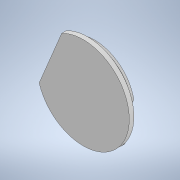
# Autodesk Inventor part: cap2
Saved by Autodesk Inventor 2020 (Build 240168000, 168)
## iProperties
Created: 2022-10-19
Part Number: cap2
Material: Типовые
Document SubType Name: Modeling
Designer: zigma
Density: 1 g/cm^3
Appearance: По умолчанию
Author: zigma
Autodesk Inventor part; units mm, degrees
ref_plane "YZ Plane" through (0, 0, 0) normal (1, 0, 0) x (0, 1, 0)
ref_plane "XZ Plane" through (0, 0, 0) normal (0, 1, 0) x (-1, 0, 0)
ref_plane "XY Plane" through (0, 0, 0) normal (0, 0, 1) x (1, 0, 0)
sketch "Эскиз1" plane through (0, 0, 0) normal (0, 0, 1) x (1, 0, 0)
  line L0 (-14.0097, -7.3348) -> (-16.3175, -6.3736)
  line L1 (-16.3175, -6.3736) -> (-14.0097, -7.3348)
  line L2 (17.7899, 2.7423) -> (-9.8124, 2.7423)
  line L3 (-14.0097, -7.3348) -> (-9.8124, 2.7423)
  line L4 (-9.8124, 2.7423) -> (17.7899, 2.7423)
  line L5 (-16.3175, -6.3736) -> (-6.7051, 16.7046)
  line L6 (-16.3175, -6.3736) -> (-6.7051, 16.7046)
  line L7 (-14.0257, -14.2577) -> (-10.5192, -14.2577)
  line L8 (-14.0257, -14.2577) -> (-10.5192, -14.2577)
  line L9 (-10.5192, -14.2577) -> (-10.5192, -12.2577)
  line L10 (-10.5192, -14.2577) -> (-10.5192, -12.2577)
  line L11 (-10.5192, -12.2577) -> (-12.5192, -12.2577)
  line L12 (-10.5192, -12.2577) -> (-12.5192, -12.2577)
  line L13 (-12.5192, -12.2577) -> (-12.5192, -10.2577)
  line L14 (-12.5192, -12.2577) -> (-12.5192, -10.2577)
  line L15 (-12.5192, -10.2577) -> (-9.4474, -10.2577)
  line L16 (-12.5192, -10.2577) -> (-9.4474, -10.2577)
  line L17 (-9.4474, -10.2577) -> (-6.5, 0.7423)
  line L18 (-9.4474, -10.2577) -> (-6.5, 0.7423)
  line L19 (-6.5, 0.7423) -> (6.5, 0.7423)
  line L20 (-6.5, 0.7423) -> (6.5, 0.7423)
  line L21 (9.4474, -10.2577) -> (12.5192, -10.2577)
  line L22 (6.5, 0.7423) -> (9.4474, -10.2577)
  line L23 (9.4474, -10.2577) -> (12.5192, -10.2577)
  line L24 (12.5192, -10.2577) -> (12.5192, -12.2577)
  line L25 (12.5192, -10.2577) -> (12.5192, -12.2577)
  line L26 (10.5192, -12.2577) -> (10.5192, -14.2577)
  line L27 (12.5192, -12.2577) -> (10.5192, -12.2577)
  line L28 (10.5192, -12.2577) -> (10.5192, -14.2577)
  line L29 (10.5192, -14.2577) -> (14.0257, -14.2577)
  arc A0 (17.7899, 2.7423) -> (-6.7051, 16.7046) centre (0, 0) ccw
  arc A1 (17.7899, 2.7423) -> (-6.7051, 16.7046) centre (0, 0) ccw
  arc A2 (17.5551, 2.9423) -> (-6.5528, 16.5499) centre (0, 0) ccw
  line L30 (17.5551, 2.9423) -> (-9.9457, 2.9423)
  line L31 (-14.1174, -7.0733) -> (-9.9457, 2.9423)
  line L32 (-16.056, -6.2659) -> (-6.5528, 16.5499)
  line L33 (-14.1174, -7.0733) -> (-16.056, -6.2659)
  arc A3 (-14.0257, -14.2577) -> (14.0257, -14.2577) centre (0, 0) ccw
  line L34 (13.5283, -14.4577) -> (10.3192, -14.4577)
  line L35 (10.3192, -12.0577) -> (10.3192, -14.4577)
  line L36 (12.3192, -12.0577) -> (10.3192, -12.0577)
  line L37 (12.3192, -10.4577) -> (12.3192, -12.0577)
  line L38 (9.294, -10.4577) -> (12.3192, -10.4577)
  line L39 (6.3465, 0.5423) -> (9.294, -10.4577)
  line L40 (-6.3465, 0.5423) -> (6.3465, 0.5423)
  line L41 (-9.294, -10.4577) -> (-6.3465, 0.5423)
  line L42 (-12.3192, -10.4577) -> (-9.294, -10.4577)
  line L43 (-12.3192, -12.0577) -> (-12.3192, -10.4577)
  line L44 (-10.3192, -12.0577) -> (-12.3192, -12.0577)
  line L45 (-10.3192, -14.4577) -> (-10.3192, -12.0577)
  line L46 (-14.0257, -14.4577) -> (-10.3192, -14.4577)
  line L47 (10.3192, -14.4577) -> (13.8194, -14.4577)
  point P0 (-13.8194, -14.4577)
  dimension "d9" = 0.2
  dimension "d10" = 0.2
  dimension "d11" = 0.2
  dimension "d12" = 0.2
  dimension "d13" = 0.2
  dimension "d15" = 0.2
  dimension "d16" = 0.2
  dimension "d17" = 0.2
  dimension "d18" = 0.2
  dimension "d19" = 0.2
  dimension "d20" = 0.2
  dimension "d21" = 0.2
  dimension "d22" = 0.2
  dimension "d23" = 0.2
  dimension "d24" = 0.2
  dimension "d25" = 0.2
  dimension "d26" = 0.2
  dimension "d27" = 3.5064
  dimension "d28" = 2
  dimension "d29" = 2
  dimension "d30" = 2
  dimension "d31" = 3.0718
  dimension "d32" = 11
  dimension "d33" = 13
  dimension "d34" = 11
  dimension "d35" = 3.0718
  dimension "d36" = 2
  dimension "d37" = 2
  dimension "d38" = 2
  dimension "d39" = 3.5064
  dimension "d40" = 20
  dimension "d41" = 2
  dimension "d42" = 0.2
  constraints: 97 end point, 16 parallel, 9 point on circle, 8 perpendicular, 7 collinear, 4 centre point, 2 horizontal, 2 point on line, 1 coincident, 1 concentric
  measures "d9" radial gap between concentric circles of A0 A2
  measures "d10" distance between parallel lines of L2 L30
  measures "d11" distance between parallel lines of L3 L31
  measures "d12" distance between parallel lines of L5 L32
  measures "d13" distance between parallel lines of L0 L33
  measures "d15" distance between parallel lines of L28 L35
  measures "d16" distance between parallel lines of L27 L36
  measures "d17" distance between parallel lines of L25 L37
  measures "d18" distance between parallel lines of L21 L38
  measures "d19" distance between parallel lines of L22 L39
  measures "d20" distance between parallel lines of L19 L40
  measures "d21" distance between parallel lines of L17 L41
  measures "d22" distance between parallel lines of L15 L42
  measures "d23" distance between parallel lines of L13 L43
  measures "d24" distance between parallel lines of L12 L44
  measures "d25" distance between parallel lines of L9 L45
  measures "d26" distance between parallel lines of L7 L46
  measures "d27" distance of L28.end L29.end
  measures "d28" distance of L27.end L28.end
  measures "d29" distance of L25.end L27.end
  measures "d30" distance of L21.end L25.end
  measures "d31" distance of L22.end L21.end
  measures "d32" vertical distance of L19.end L22.end
  measures "d33" distance of L17.end L19.end
  measures "d34" vertical distance of L17.start L17.end
  measures "d35" distance of L15.start L17.start
  measures "d36" distance of L12.end L15.start
  measures "d37" distance of L12.start L12.end
  measures "d38" distance of L7.end L12.start
  measures "d39" distance of L7.start L7.end
  measures "d40" radius of A3
  measures "d41" distance between parallel lines of L2 L19
  measures "d42" distance between parallel lines of L29 L34
extrude "Выдавливание1" add sketch "Эскиз1" along normal blind 3 contours L46 L45 L44 L43 L42 L41 L40 L39 L38 L37 L36 L35 L34 L47 A3 | L30 L31 L33 L32 A2
sketch "Эскиз3" plane through (0, 0, 3) normal (0, 0, 1) x (1, 0, 0)
  arc A0 (-19.1284, -5.8399) -> (-9.3269, 17.692) centre (0, 0) ccw
  arc A1 (-14.0257, -14.2577) -> (14.0257, -14.2577) centre (0, 0) ccw projected
  line L0 (-19.1284, -5.8399) -> (-9.3269, 17.692)
  line L1 (-6.5528, 16.5499) -> (-16.056, -6.2659) projected
  dimension "d43" = 3
  constraints: 2 end point, 2 point on circle, 1 centre point, 1 coincident, 1 concentric, 1 parallel
  measures "d43" distance between parallel lines of L1 L0
extrude "Выдавливание3" add sketch "Эскиз3" along normal blind 2
chamfer "Фаска2" distance 0.5 angle 70 5 edges at (3.8047, 2.9423, 0) (8.7496, 15.5011, 0) (-11.3044, 5.142, 0) (-15.0867, -6.6696, 0) (-12.0316, -2.0655, 0) measured on face at (8.027, 4.2106, 0)
chamfer "Фаска3" distance 0.5 angle 70 12 edges at (7.8203, -4.9577, 0) (10.8066, -10.4577, 0) (12.3192, -11.2577, 0) (11.3192, -12.0577, 0) (10.3192, -13.2577, 0) (11.9238, -14.4577, 0) (-12.0693, -14.4577, 0) (-10.3192, -13.2577, 0) (-11.3192, -12.0577, 0) (-10.8066, -10.4577, 0) (-7.8203, -4.9577, 0) (0, 0.5423, 0) measured on face at (-1.9545, -6.8341, 0) measured on face at (1.7704, -6.791, 0) measured on face at (2.1155, -6.791, 0)
